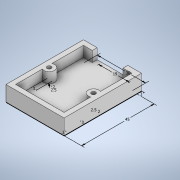
# Autodesk Inventor part: dongle shell
Saved by Autodesk Inventor 2020.3 (Build 243373010, 373A)
## iProperties
Created: 2020-10-03
Part Number: dongle shell
Material: Generic
Document SubType Name: Modeling
Designer: joesp
Density: 1 g/cm^3
Appearance: Default
Author: joesp
Autodesk Inventor part; units mm, degrees
ref_plane "YZ Plane" through (0, 0, 0) normal (1, 0, 0) x (0, 1, 0)
ref_plane "XZ Plane" through (0, 0, 0) normal (0, 1, 0) x (-1, 0, 0)
ref_plane "XY Plane" through (0, 0, 0) normal (0, 0, 1) x (1, 0, 0)
sketch "Sketch1" plane through (0, 0, 0) normal (0, 1, 0) x (-1, 0, 0)
  line L0 (0, 0) -> (30, 0)
  line L1 (30, 0) -> (30, 45)
  line L2 (30, 45) -> (0, 45)
  line L3 (0, 45) -> (0, 0)
  line L4 (33, 0) -> (-3, 0)
  line L5 (-3, 0) -> (-3, 45)
  line L6 (-3, 45) -> (33, 45)
  line L7 (33, 45) -> (33, 0)
  line L8 (30, 45) -> (0, 45)
  line L9 (0, 45) -> (0, 42)
  line L10 (0, 42) -> (30, 42)
  line L11 (30, 42) -> (30, 45)
  line L12 (24.5, 0) -> (5.5, 0)
  line L13 (5.5, 0) -> (5.5, -3)
  line L14 (5.5, -3) -> (24.5, -3)
  line L15 (24.5, -3) -> (24.5, 0)
  line L16 (24.5, 0) -> (33, 0)
  line L17 (33, 0) -> (33, -3)
  line L18 (33, -3) -> (24.5, -3)
  line L19 (24.5, -3) -> (24.5, 0)
  line L20 (5.5, 0) -> (-3, 0)
  line L21 (-3, 0) -> (-3, -3)
  line L22 (-3, -3) -> (5.5, -3)
  line L23 (5.5, -3) -> (5.5, 0)
  circle A0 centre (28.75, 22.5) radius 1.25
  circle A1 centre (1.25, 22.5) radius 1.25
  circle A2 centre (28.75, 22.5) radius 3.25
  circle A3 centre (1.25, 22.5) radius 3.25
  point P0 (33, 22.5)
  point P1 (33, 22.5)
  point P2 (5.5, 0)
  point P3 (30, 19.5)
  point P4 (0, 19.5)
  point P5 (0, 25.5)
  point P6 (30, 25.5)
  dimension "d0" = 3
  dimension "d1" = 3
  dimension "d2" = 30
  dimension "d3" = 45
  dimension "d4" = 3
  dimension "d5" = 19
  dimension "d6" = 3
  dimension "d7" = 2.5
  dimension "d8" = 2.5
  dimension "d9" = 2
  dimension "d10" = 2
  constraints: 48 end point, 12 parallel, 6 horizontal, 6 perpendicular, 4 centre point, 4 point on line, 3 coincident, 2 horizontal alignment, 2 tangent, 1 collinear, 1 midpoint
  measures "d0" distance between parallel lines of L1 L7
  measures "d1" distance between parallel lines of L5 L3
  measures "d2" distance of L0.start L0.end
  measures "d3" distance of L4.end L5.end
  measures "d4" distance from line of L2 L9.end
  measures "d5" distance of L13.end L14.end
  measures "d6" distance of L4.end L21.end
  measures "d7" diameter of A0
  measures "d8" diameter of A1
  measures "d9" radial gap between concentric circles of A2 A0
  measures "d10" radial gap between concentric circles of A3 A1
extrude "Extrusion1" add sketch "Sketch1" along normal blind 3
extrude "Extrusion2" add sketch "Sketch1" along normal blind 9.5 contours L4 L5 L6 L3 A3 | L0 L13 L22 L21 L4 | A3 L3 | L3 A3 | L0 L4 L17 L18 L15 | L1 A2 L6 L7 L4 | L3 L2 L1 L10 | A2 L1 | L1 A2
body "Solid1"
